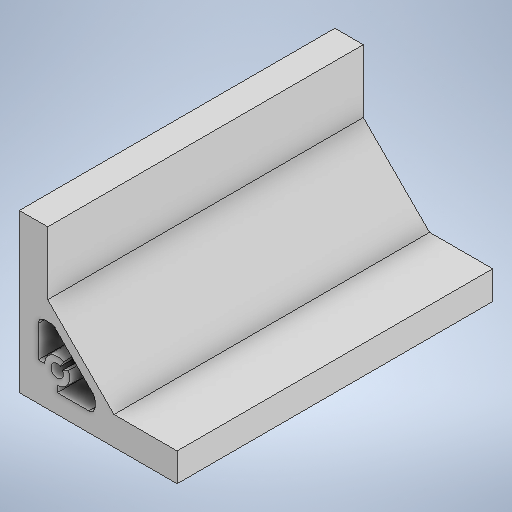
# Autodesk Inventor part: Profile_50x50x9
Saved by Autodesk Inventor 2025.2 (Build 292293000, 293)
## iProperties
Created: 2025-04-05
Part Number: Profile_50x50x9
Material: Generic
Document SubType Name: Modeling
Designer: kenne
Density: 1 g/cm^3
Appearance: Default
Author: kenne
Autodesk Inventor part; units mm, degrees
ref_plane "YZ Plane" through (0, 0, 0) normal (1, 0, 0) x (0, 1, 0)
ref_plane "XZ Plane" through (0, 0, 0) normal (0, 1, 0) x (-1, 0, 0)
ref_plane "XY Plane" through (0, 0, 0) normal (0, 0, 1) x (1, 0, 0)
sketch "Sketch1" plane through (0, 0, 0) normal (0, 0, 1) x (1, 0, 0)
  line L0 (-25, 0) -> (25, 0)
  line L1 (-25, 0) -> (-25, 50)
  line L2 (-25, 50) -> (-16, 50)
  line L3 (-16, 50) -> (-16, 30)
  line L4 (25, 9) -> (25, 0)
  line L5 (5, 9) -> (25, 9)
  line L6 (-16, 30) -> (5, 9)
  line L7 (-36, 0) -> (-36, 12) construction
  line L8 (-25, -11) -> (-13, -11) construction
  circle A0 centre (-13, 12) radius 2 construction
  line L9 (-25, 0) -> (-36, 0) construction
  line L10 (-25, 0) -> (-25, -11) construction
  line L11 (-19, 12) -> (-19, 22)
  line L12 (-13, 6) -> (-3, 6)
  line L13 (-13.6569, 23.4142) -> (-1.5858, 11.3431)
  line L14 (-19, 12) -> (-17, 12)
  circle A1 centre (-13, 12) radius 4 construction
  arc A2 (-11, 15.4641) -> (-17, 12) centre (-13, 12) ccw
  line L15 (-13, 6) -> (-13, 8)
  arc A3 (-13, 8) -> (-9.4446, 13.8328) centre (-13, 12) ccw
  line L16 (-11, 15.4641) -> (-12, 13.7321)
  arc A4 (-12, 13.7321) -> (-11.2679, 13) centre (-13, 12) ccw
  line L17 (-9.4446, 13.8328) -> (-11.2679, 13)
  line L18 (-17, 24) -> (-15.0711, 24)
  line L19 (-1, 9.9289) -> (-1, 8)
  arc A5 (-17, 24) -> (-19, 22) centre (-17, 22) ccw
  arc A6 (-13.6569, 23.4142) -> (-15.0711, 24) centre (-15.0711, 22) ccw
  arc A7 (-1, 9.9289) -> (-1.5858, 11.3431) centre (-3, 9.9289) ccw
  arc A8 (-3, 6) -> (-1, 8) centre (-3, 8) ccw
  point P0 (0, 0)
  point P1 (0, 0)
  point P2 (-19, 24)
  point P3 (-1, 6)
  point P4 (-14.2426, 24)
  point P5 (-1, 10.7574)
  point P6 (-15, 15.4641)
  dimension "d0" = 50
  dimension "d1" = 0
  dimension "expessura" = 9
  dimension "secondary" = 20
  dimension "d4" = 9
  dimension "d5" = 20
  dimension "d6" = 12
  dimension "d7" = 36
  dimension "d8" = 12
  dimension "d9" = 11
  dimension "d10" = 4
  dimension "inner_width" = 6
  dimension "d12" = 6
  dimension "d13" = 12
  dimension "d14" = 12
  dimension "d15" = 3
  dimension "d16" = 2
  dimension "d17" = 2
  dimension "d18" = 3.4641
  dimension "d19" = 117.271
  dimension "d21" = 1.7321
  dimension "d22" = 1.8234
  dimension "d23" = 2
  constraints: 40 end point, 20 point on circle, 11 tangent, 9 centre point, 8 horizontal, 8 point on line, 8 vertical, 4 equal radius, 3 horizontal alignment, 3 vertical alignment, 2 coincident, 1 midpoint, 1 parallel, 1 perpendicular
  measures "d0" distance of L0.start L0.end
  measures "d1" distance from line of L0 point (0, 0)
  measures "expessura" distance of L1.end L2.end
  measures "secondary" distance of L2.end L3.end
  measures "d4" distance of L4.start L0.end
  measures "d5" distance of L5.start L4.start
  measures "d6" distance of L7.start L7.end
  measures "d7" distance from line of point (0, 0) L7
  measures "d8" distance of L8.start L8.end
  measures "d9" distance from line of point (0, 0) L8
  measures "d10" diameter of A0
  measures "inner_width" distance between parallel lines of L11 L1
  measures "d12" distance between parallel lines of L0 L12
  measures "d13" distance of L11.start point (-19, 24)
  measures "d14" distance of L12.start point (-1, 6)
  measures "d15" distance between parallel lines of L13 L6
  measures "d16" distance of L11.start L14.end
  measures "d17" radial gap between concentric circles of A0 A1
  measures "d18" vertical distance of A0.centre point (-15, 15.464)
  measures "d21" vertical distance of L16.start L16.end
  measures "d22" horizontal distance of L17.start L17.end
  measures "d23" radius of A5
extrude "Extrusion1" add sketch "Sketch1" along normal mid plane 100
equation "\"d4\" = expessura"
equation "\"d5\" = secondary"
equation "\"d12\" = inner_width"
body "Solid1"
